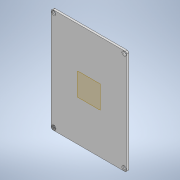
# Autodesk Inventor part: Bottom_lid
Saved by Autodesk Inventor 2022 (Build 260153000, 153)
## iProperties
Created: 2021-01-26
Part Number: Bottom_lid
Material: Generic
Document SubType Name: Modeling
Designer: simen
Density: 1 g/cm^3
Appearance: Default
Author: simen
## iProperties of the stored document Bottom_lid_3DPrint.ipt
Created: 2021-12-09
Part Number: Bottom_lid_3DPrint
Material: Generic
Document SubType Name: Modeling
Designer: simen
Density: 1 g/cm^3
Appearance: Default
Author: simen
Autodesk Inventor part; units mm, degrees
ref_plane "YZ Plane" through (0, 0, 0) normal (1, 0, 0) x (0, 1, 0)
ref_plane "XZ Plane" through (0, 0, 0) normal (0, 1, 0) x (-1, 0, 0)
ref_plane "XY Plane" through (0, 0, 0) normal (0, 0, 1) x (1, 0, 0)
ref_plane "Work Plane3" through (0, 0, 0) normal (0, 0, 1) x (1, 0, 0)
sketch "Sketch1" plane through (0, 0, 0) normal (0, 0, 1) x (1, 0, 0)
  line L0 (37, 49) -> (37, -49) projected
  arc A0 (37, 49) -> (35, 51) centre (35, 49) ccw projected
  line L1 (-35, 51) -> (35, 51) projected
  line L2 (-37, -49) -> (-37, 49) projected
  arc A1 (-35, 51) -> (-37, 49) centre (-35, 49) ccw projected
  arc A2 (-37, -49) -> (-35, -51) centre (-35, -49) ccw projected
  line L3 (35, -51) -> (-35, -51) projected
  arc A3 (35, -51) -> (37, -49) centre (35, -49) ccw projected
  arc A4 (36.5, 49) -> (35, 50.5) centre (35, 49) ccw
  line L4 (36.5, 49) -> (36.5, -49)
  arc A5 (35, -50.5) -> (36.5, -49) centre (35, -49) ccw
  line L5 (35, -50.5) -> (-35, -50.5)
  arc A6 (-36.5, -49) -> (-35, -50.5) centre (-35, -49) ccw
  line L6 (-36.5, -49) -> (-36.5, 49)
  arc A7 (-35, 50.5) -> (-36.5, 49) centre (-35, 49) ccw
  line L7 (-35, 50.5) -> (35, 50.5)
  circle A8 centre (34, 48) radius 1.5 projected
  circle A9 centre (34, -48) radius 1.5 projected
  circle A10 centre (-34, -48) radius 1.5 projected
  circle A11 centre (34, 48) radius 1.6
  circle A12 centre (34, -48) radius 1.6
  circle A13 centre (-34, -48) radius 1.6
  circle A14 centre (-34, 48) radius 1.6
  point P0 (0, 0)
  point P1 (-33, 42)
  dimension "d0" = 0.5
  dimension "d1" = 3.2
  dimension "d2" = 3.2
  dimension "d3" = 3.2
  dimension "d7" = 2.5
  dimension "d8" = 2.5
  dimension "d11" = 3.2
  dimension "d12" = 2.5
  dimension "d13" = 2.5
  constraints: 8 centre point, 8 end point, 8 point on circle, 3 coincident, 7 other
  measures "d0" distance between parallel lines of L1 L7
  measures "d1" diameter of A11
  measures "d2" diameter of A12
  measures "d3" diameter of A13
  measures "d7" distance from line of L7 A8.centre
  measures "d8" distance from line of L4 A8.centre
  measures "d11" diameter of A14
  measures "d12" distance from line of L7 A14.centre
  measures "d13" distance from line of L6 A14.centre
extrude "Extrusion1" add sketch "Sketch1" against normal blind 2 contours L4 A5 L5 A6 L6 A7 L7 A4
chamfer "Chamfer1" distance 0.5 angle 45 4 edges at (32.4, 48, 0) (32.4, -48, 0) (-35.6, -48, 0) (-35.6, 48, 0)
body "Solid1"
